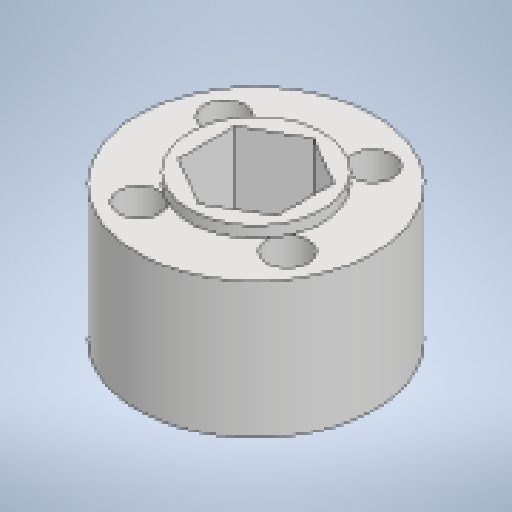
# Autodesk Inventor part: GoBilda Mech Hub 0500 Hex Spacer  inserts V2
Saved by Autodesk Inventor 2023 (Build 270158000, 158)
## iProperties
Created: 2021-12-21
Part Number: GoBilda Mech Hub 0500 Hex Spacer  inserts V2
Material: Generic
Document SubType Name: Modeling
Designer: TakeHomePC
Density: 1 g/cm^3
Appearance: Default
Author: TakeHomePC
Autodesk Inventor part; units mm, degrees
ref_plane "YZ Plane" through (0, 0, 0) normal (1, 0, 0) x (0, 1, 0)
ref_plane "XZ Plane" through (0, 0, 0) normal (0, 1, 0) x (-1, 0, 0)
sketch "Sketch1" plane through (0, 0, 0) normal (0, 1, 0) x (-1, 0, 0)
  circle A0 centre (9.798, -5.6569) radius 3.4
  circle A1 centre (0, 0) radius 15.739
  line L0 (0, -7.5575) -> (-6.545, -3.7788)
  line L1 (-6.545, -3.7788) -> (-6.545, 3.7788)
  line L2 (-6.545, 3.7788) -> (0, 7.5575)
  line L3 (0, 7.5575) -> (6.545, 3.7788)
  line L4 (6.545, 3.7788) -> (6.545, -3.7788)
  line L5 (6.545, -3.7788) -> (0, -7.5575)
  circle A2 centre (5.6569, 9.798) radius 3.4
  circle A3 centre (-9.798, 5.6569) radius 3.4
  circle A4 centre (-5.6569, -9.798) radius 3.4
  circle A5 centre (5.6569, 9.798) radius 1.86 projected
  circle A6 centre (0, 0) radius 8.8161
  circle A7 centre (5.6569, 9.798) radius 2.7
  circle A8 centre (-9.798, 5.6569) radius 2.7
  circle A9 centre (-5.6569, -9.798) radius 2.7
  circle A10 centre (9.798, -5.6569) radius 2.7
  line L6 (-3.6579, 5.4456) -> (-8.2517, 13.4024)
  line L7 (-8.1837, 13.2847) -> (-7.413, 13.7297)
  line L8 (-7.481, 13.8474) -> (-2.8871, 5.8906)
  line L9 (0.9331, -2.5201) -> (-7.413, 13.7297) construction
  line L10 (-8.2574, 13.3989) -> (1.7159, -2.0681) construction
  point P0 (0, 0)
  point P1 (-3.2725, 5.6681)
  point P2 (-4.0171, 7.8477)
  point P3 (-7.4748, 13.8507)
  point P4 (-8.2577, 13.3988)
  point P5 (-4.7878, 7.4027)
  dimension "d0" = 31.478
  dimension "d3" = 13.09
  dimension "d4" = 6.8
  dimension "d7" = 360
  dimension "d13" = 5.4
  dimension "d16" = 360
  constraints: 22 end point, 10 centre point, 7 point on line, 5 coincident, 3 point on circle, 2 perpendicular, 1 midpoint, 1 parallel, 31 other
  measures "d0" diameter of A1
  measures "d3" distance between parallel lines of L4 L1
  measures "d4" diameter of A0
  measures "d13" diameter of A7
extrude "Extrusion1" add sketch "Sketch1" along normal blind 18 contours A0 A6 A2 L8 A1 L6 A3 A4 | A0 A6 A4 A3 L6 L2 L1 L0 L5 L4 L3 L8 A2 | L8 L2 L6 A6 | A6 L6 L7 L8 | L7 L6 A1 L8
ref_plane "Work Plane1" through (-24.2096, 24.4273, -24.2096) normal (0, 1, 0) x (0.0853, 0, 0.9964)
extrude "Extrusion2" add sketch "Sketch1" along normal blind 1.5 from surface at 18 contours A6 A10 A0 | A0 A6 A4 A3 L6 L2 L1 L0 L5 L4 L3 L8 A2 | A6 A10 | A6 A9 A4 | A2 A6 A7 | A6 A9 | A7 A6 | A6 A8 A3 | L8 L2 L6 A6 | A6 A8 picked at (7.7135, -3.2903) picked at (7.577, -4.2584) picked at (-3.2903, -7.7135) picked at (5.035, 6.7062) picked at (-4.2584, -7.577) picked at (4.4327, 7.4764) picked at (-6.8562, 4.5301) picked at (-7.577, 4.2584)
extrude "Extrusion4" add sketch "Sketch1" against normal blind 6.5 from surface at 18 contours A0 A6 A10 | A6 A10 A0 | A6 A9 A4 | A4 A6 A9 | A6 A7 A2 | A2 A6 A7 | A6 A8 A3 | A3 A6 A8
extrude "Extrusion5" cut sketch "Sketch1" against normal blind 0.5 from surface at 18 contours A0 A6 A10 | A0 A6 A2 L8 A1 L6 A3 A4 | A10 A6 | A4 A6 A9 | A6 A7 A2 | A9 A6 | A6 A7 | A3 A6 A8 | A6 L6 L7 L8 | A8 A6 | L7 L6 A1 L8 | A5 picked at (12.9069, -5.176) picked at (10.5068, -6.3265) picked at (-2.5233, -10.0696) picked at (8.7688, 9.3298) picked at (-6.0238, -10.6855) picked at (8.051, 10.0123) picked at (-12.6093, 4.2453) picked at (-10.5428, 6.2692)
extrude "Extrusion6" cut sketch "Sketch1" along normal through all contours L7 L6 A1 L8
extrude "Extrusion7" cut sketch "Sketch1" against normal blind 0.5 from surface at 17.5 contours A6 L6 L7 L8
body "Solid1"
